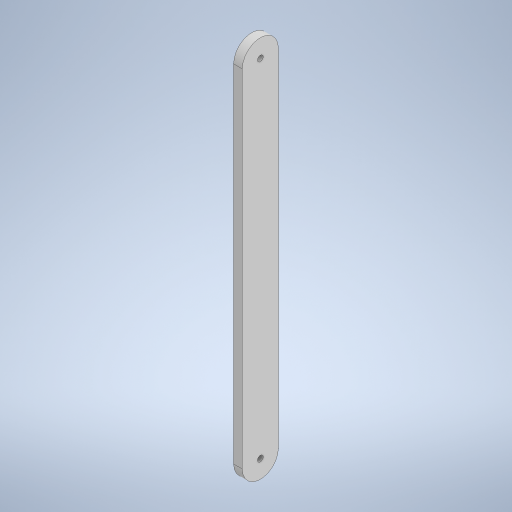
# Autodesk Inventor part: Vertical
Saved by Autodesk Inventor 2024 (Build 280153000, 153)
## iProperties
Created: 2024-03-09
Part Number: Vertical
Material: Generic
Document SubType Name: Modeling
Designer: ddcos
Density: 1 g/cm^3
Appearance: Default
Author: ddcos
Autodesk Inventor part; units mm, degrees
ref_plane "YZ Plane" through (0, 0, 0) normal (1, 0, 0) x (0, 1, 0)
ref_plane "XZ Plane" through (0, 0, 0) normal (0, 1, 0) x (-1, 0, 0)
ref_plane "XY Plane" through (0, 0, 0) normal (0, 0, 1) x (1, 0, 0)
sketch "Sketch1" plane through (0, 0, 0) normal (0, 0, 1) x (1, 0, 0)
  line L0 (0, 0) -> (-25, 0)
  line L1 (-25, 0) -> (-25, 265)
  line L2 (-25, 265) -> (0, 265)
  line L3 (0, 265) -> (0, 0)
  dimension "d0" = 265
  dimension "d1" = 25
  constraints: 8 end point, 2 parallel, 1 horizontal, 1 perpendicular
  measures "d0" distance of L2.end L0.start
  measures "d1" distance of L0.start L0.end
extrude "Extrusion1" add sketch "Sketch1" along normal blind 25
sketch "Sketch2" plane through (0, 0, 0) normal (1, 0, 0) x (0, 0, -1)
  circle A0 centre (-12.5, 12.5) radius 12.5
  line L0 (0, 0) -> (-25, 0) projected
  circle A1 centre (-12.5, 12.5) radius 2
  circle A2 centre (-12.5, 252.5) radius 12.5
  line L1 (0, 265) -> (-25, 265) projected
  circle A3 centre (-12.5, 252.5) radius 2
  line L2 (0, 0) -> (0, 265) projected
  line L3 (-25, 0) -> (-25, 265) projected
  point P0 (-12.5, 0)
  point P1 (-25, 252.5)
  point P2 (-12.5, 265)
  point P3 (0, 252.5)
  point P4 (-25, 12.5)
  point P5 (-12.5, 0)
  point P6 (0, 12.5)
  dimension "d4" = 25
  dimension "d5" = 12.5
  dimension "d6" = 4
  dimension "d7" = 25
  dimension "d8" = 12.5
  dimension "d9" = 4
  dimension "d10" = 12.5
  dimension "d11" = 12.5
  constraints: 4 centre point, 2 coincident, 1 midpoint
  measures "d4" diameter of A0
  measures "d5" distance of point (-12.5, 0) A0.centre
  measures "d6" diameter of A1
  measures "d7" diameter of A2
  measures "d8" distance from line of L1 A2.centre
  measures "d9" diameter of A3
  measures "d10" distance from line of L2 A2.centre
  measures "d11" distance from line of L2 A0.centre
extrude "Extrusion2" cut sketch "Sketch2" against normal blind 25 contours L2 L0 A0 | A0 L0 L3 | A2 L1 L2 | L3 L1 A2 | A1 | A3
sketch "Sketch3" plane through (0, 0, 25) normal (0, 0, 1) x (1, 0, 0)
  line L0 (-25, 265) -> (0, 265) projected
  line L1 (0, 0) -> (-19, 0)
  line L2 (-19, 0) -> (-19, 265)
  line L3 (-19, 265) -> (0, 265)
  line L4 (0, 265) -> (0, 0)
  point P0 (0, 265)
  dimension "d14" = 19
  constraints: 8 end point, 2 parallel, 1 horizontal, 1 perpendicular, 1 point on line
  measures "d14" distance of L2.end L3.end
extrude "Extrusion3" cut sketch "Sketch3" against normal blind 100
body "Solid1"
